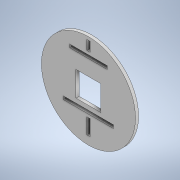
# Autodesk Inventor part: Slider_1
Saved by Autodesk Inventor 2022.2 (Build 262287010, 287A)
## iProperties
Created: 2023-12-11
Part Number: Slider_1
Material: Generisch
Document SubType Name: Modeling
Designer: ppovolni
Density: 1 g/cm^3
Appearance: Vorgabe
Author: ppovolni
Autodesk Inventor part; units mm, degrees
ref_plane "YZ Plane" through (0, 0, 0) normal (1, 0, 0) x (0, 1, 0)
ref_plane "XZ Plane" through (0, 0, 0) normal (0, 1, 0) x (-1, 0, 0)
ref_plane "XY Plane" through (0, 0, 0) normal (0, 0, 1) x (1, 0, 0)
sketch "Skizze1" plane through (0, 0, 0) normal (0, 0, 1) x (1, 0, 0)
  circle A0 centre (0, 0) radius 80 construction
  circle A1 centre (0, 0) radius 76 construction
  circle A2 centre (0, 0) radius 75.5
  line L0 (-15, 25) -> (15, 25) construction
  line L1 (15, 25) -> (15, -25) construction
  line L2 (15, -25) -> (-15, -25) construction
  line L3 (-15, -25) -> (-15, 25) construction
  line L4 (-15, 25) -> (15, -25) construction
  line L5 (15, 25) -> (-15, -25) construction
  line L6 (-40.1, -27) -> (40.1, -27)
  line L7 (40.1, -27) -> (40.1, -32.2)
  line L8 (40.1, -32.2) -> (-40.1, -32.2)
  line L9 (-40.1, -32.2) -> (-40.1, -27)
  line L10 (-2.6, -32.2) -> (2.6, -32.2)
  line L11 (-30.1, 45) -> (30.1, 45)
  line L12 (30.1, 45) -> (30.1, 50.2)
  line L13 (30.1, 50.2) -> (-30.1, 50.2)
  line L14 (-30.1, 50.2) -> (-30.1, 45)
  line L15 (-2.6, -37.2) -> (2.6, -37.2)
  line L16 (2.6, -37.2) -> (2.6, -62.4)
  line L17 (2.6, -62.4) -> (-2.6, -62.4)
  line L18 (-2.6, -62.4) -> (-2.6, -37.2)
  line L19 (-20, 20) -> (20, 20)
  line L20 (20, 20) -> (20, -20)
  line L21 (20, -20) -> (-20, -20)
  line L22 (-20, -20) -> (-20, 20)
  line L23 (-20, 20) -> (20, -20) construction
  line L24 (20, 20) -> (-20, -20) construction
  line L25 (-2.6, 70.4) -> (2.6, 70.4)
  line L26 (2.6, 70.4) -> (2.6, 55.2)
  line L27 (2.6, 55.2) -> (-2.6, 55.2)
  line L28 (-2.6, 55.2) -> (-2.6, 70.4)
  point P0 (0, -32.2)
  point P1 (0, -32.2)
  point P2 (0, -32.2)
  point P3 (0, 45)
  point P4 (0, -37.2)
  dimension "d0" = 160
  dimension "d1" = 4
  dimension "d2" = 0.5
  dimension "d6" = 30
  dimension "d7" = 50
  dimension "d8" = 2
  dimension "d9" = 80.2
  dimension "d10" = 5.2
  dimension "d13" = 5.2
  dimension "d14" = 60.2
  dimension "d15" = 5.2
  dimension "d16" = 45
  dimension "d17" = 5.2
  dimension "d18" = 25.2
  dimension "d19" = 5
  dimension "d20" = 40
  dimension "d21" = 5
  dimension "d22" = 15.2
  constraints: 58 end point, 12 parallel, 8 midpoint, 7 horizontal, 6 perpendicular, 5 vertical alignment, 4 coincident, 3 centre point, 2 equal length, 1 collinear, 1 point on line
  measures "d0" diameter of A0
  measures "d1" radial gap between concentric circles of A1 A0
  measures "d2" radial gap between concentric circles of A2 A1
  measures "d6" distance of L0.start L0.end
  measures "d7" distance of L2.end L0.start
  measures "d8" distance between parallel lines of L6 L2
  measures "d9" distance of L7.end L8.end
  measures "d10" distance of L8.end L6.start
  measures "d13" distance of L11.end L12.end
  measures "d14" distance of L12.end L13.end
  measures "d15" distance of L13.end L11.start
  measures "d16" distance from line of point (0, 0) L11
  measures "d17" distance of L16.end L17.end
  measures "d18" distance of L17.end L15.start
  measures "d19" distance between parallel lines of L15 L8
  measures "d20" distance of L19.start L19.end
  measures "d21" distance between parallel lines of L13 L27
  measures "d22" distance of L25.end L26.end
extrude "Extrusion1" add sketch "Skizze1" along normal blind 5
